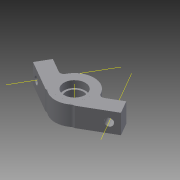
# Autodesk Inventor part: right top
Saved by Autodesk Inventor 2013 (Build 170138000, 138)
## iProperties
Created: 2012-12-31
Part Number: right top
Material: Generic
Document SubType Name: Modeling
Designer: Nico
Density: 1 g/cm^3
Author: Nico
Autodesk Inventor part; units mm, degrees
ref_plane "YZ Plane" through (0, 0, 0) normal (1, 0, 0) x (0, 1, 0)
ref_plane "XZ Plane" through (0, 0, 0) normal (0, 1, 0) x (-1, 0, 0)
sketch "Sketch1" plane through (0, 0, 0) normal (0, 0, 1) x (1, 0, 0)
  circle A0 centre (0, 0) radius 9
  circle A1 centre (0, 0) radius 15
  dimension "d0" = 18
  dimension "d3" = 30
  constraints: 2 centre point, 2 coincident
  measures "d0" diameter of A0
  measures "d3" diameter of A1
extrude "Extrusion1" add sketch "Sketch1" along normal blind 20
sketch "Sketch2" plane through (0, 0, 20) normal (0, 0, 1) x (1, 0, 0)
  circle A0 centre (0, 0) radius 9 projected
  circle A1 centre (0, 0) radius 15 projected
  circle A2 centre (0, 0) radius 11
  dimension "d6" = 22
  constraints: 1 centre point, 1 coincident
  measures "d6" diameter of A2
extrude "Extrusion2" cut sketch "Sketch2" against normal blind 7 contours A2
sketch "Sketch3" plane through (0, 0, 0) normal (0, 0, -1) x (-1, 0, 0)
  circle A0 centre (0, 0) radius 9 projected
  circle A1 centre (0, 0) radius 15 projected
  circle A2 centre (0, 0) radius 11
  dimension "d10" = 22
  constraints: 1 centre point, 1 coincident
  measures "d10" diameter of A2
extrude "Extrusion3" cut sketch "Sketch3" against normal blind 7 contours A2
sketch "Sketch4" plane through (0, 0, 20) normal (0, 0, 1) x (1, 0, 0)
  circle A0 centre (0, 0) radius 11 projected
  circle A1 centre (0, 0) radius 15 projected
  line L0 (-15, 0) -> (15, 0)
  constraints: 2 end point, 2 point on circle, 1 horizontal
ref_plane "Work Plane2" through (-15, -15, 20) normal (0, -1, 0) x (1, 0, 0)
ref_plane "Work Plane1" through (-15, 0, 20) normal (0, -1, 0) x (1, 0, 0)
sketch "Sketch5" plane through (-15, -15, 20) normal (0, -1, 0) x (1, 0, 0)
  line L0 (-0.0102, -19.9878) -> (29.9898, -19.9878)
  line L1 (29.9898, -19.9878) -> (29.9898, 0.0122)
  line L2 (29.9898, 0.0122) -> (-0.0102, 0.0122)
  line L3 (-0.0102, 0.0122) -> (-0.0102, -19.9878)
  point P0 (15, -20)
  dimension "d16" = 20
  dimension "d18" = 30
  constraints: 8 end point, 2 parallel, 1 horizontal, 1 perpendicular
  measures "d16" distance between parallel lines of L0 L2
  measures "d18" distance of L0.start L0.end
extrude "Extrusion4" add sketch "Sketch5" against normal blind 4
sketch "Sketch6" plane through (-15.0102, -15, 20.0122) normal (0, 0, 1) x (1, 0, 0)
  line L0 (30, 0) -> (0, 0) projected
  line L1 (30, 0) -> (30, 4) projected
  line L2 (0, 4) -> (30, 4) projected
  line L3 (0, 0) -> (0, 4) projected
  line L4 (0, 0) -> (-30.3109, 17.5)
  line L5 (30, 0) -> (60.3109, 17.5)
  line L6 (-30.3109, 17.5) -> (-22.8109, 30.4904)
  line L7 (-22.8109, 30.4904) -> (0.1146, 17.2544)
  line L8 (60.3109, 17.5) -> (52.8109, 30.4904)
  line L9 (52.8109, 30.4904) -> (29.8854, 17.2544)
  arc A0 (0.1146, 17.2544) -> (4.7165, 4) centre (15.0102, 15) ccw
  line L10 (0, 0) -> (15.0157, -0.0652)
  line L11 (30, 0) -> (16.4105, 0)
  arc A1 (25.3039, 4) -> (29.9041, 17.2652) centre (15.0102, 15) ccw
  arc A2 (16.4105, 0) -> (25.3039, 4) centre (15.0102, 15) ccw
  arc A3 (13.6098, 0) -> (16.4105, 0) centre (15.0102, 15) ccw
  arc A4 (4.7165, 4) -> (13.6098, 0) centre (15.0102, 15) ccw
  circle A5 centre (15.0102, 15) radius 15.0652
  dimension "d40" = 30.1304
  dimension "d21" = 30
  dimension "d22" = 30
  dimension "d23" = 35
  dimension "d24" = 35
  dimension "d25" = 90
  dimension "d26" = 90
  dimension "d27" = 15
  constraints: 16 end point, 11 point on circle, 5 centre point, 5 point on line, 4 perpendicular, 2 coincident, 3 other
  measures "d21" angle of L0 L4
  measures "d22" angle of L0 L5
  measures "d23" distance of L0.end L4.end
  measures "d24" distance of L0.start L5.end
  measures "d25" angle of L6 L7
  measures "d26" angle of L4 L6
  measures "d27" distance between parallel lines of L4 L7
extrude "Extrusion5" add sketch "Sketch6" against normal blind 20 contours L1 L2 A1 L9 L8 L5 | L4 L6 L7 A0 L2 L3
sketch "Sketch7" plane through (-45.3211, 2.5, 0.0122) normal (-0.5, -0.866, 0) x (0.866, -0.5, 0)
  circle A0 centre (9, 10) radius 3.9
  line L0 (0, 20) -> (0, 0) projected
  point P0 (40.4992, -0.0122)
  dimension "d30" = 7.8
  dimension "d39" = 9
  constraints: 1 centre point
  measures "d30" diameter of A0
  measures "d39" distance from line of L0 A0.centre
extrude "Extrusion6" cut sketch "Sketch7" against normal blind 20
sketch "Sketch8" plane through (14.9898, -15, 0.0122) normal (0.5, -0.866, 0) x (0.866, 0.5, 0)
  line L0 (35, 20) -> (35, 0) projected
  circle A0 centre (26, 10) radius 3.9
  point P0 (-5.4816, -0.0122)
  dimension "d34" = 7.8
  dimension "d36" = 9
  constraints: 1 centre point
  measures "d34" diameter of A0
  measures "d36" distance from line of A0.centre L0
extrude "Extrusion7" cut sketch "Sketch8" against normal blind 20
sketch "Sketch9" plane through (0, 0, 20) normal (0, 0, 1) x (1, 0, 0)
  circle A0 centre (0, 0) radius 11 projected
  arc A1 (10.198, -11) -> (-10.198, -11) centre (0, 0) ccw projected
  circle A2 centre (0, 0) radius 20
  dimension "d41" = 40
  constraints: 1 centre point, 1 coincident
  measures "d41" diameter of A2
extrude "Extrusion8" add sketch "Sketch9" against normal blind 20
fillet "Fillet1" radius 4 2 edges at (-13.2288, -15, 10.0061) (13.2288, -15, 10.0061)
fillet "Fillet2" radius 4 2 edges at (-19.4016, 4.8559, 10.0061) (19.399, 4.8661, 10.0061)
body "Solid1"
